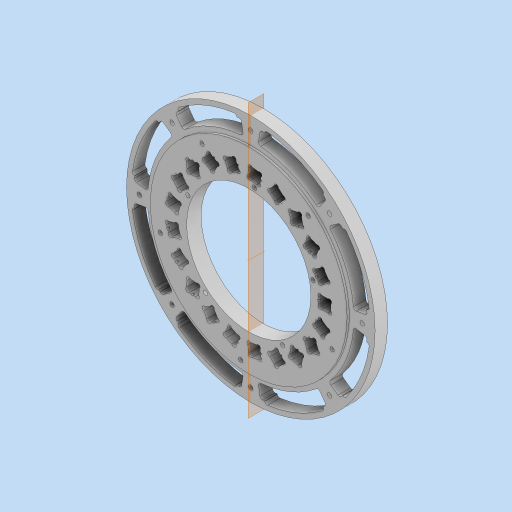
# Autodesk Inventor part: Ring_0
Saved by Autodesk Inventor 2024.2 (Build 282272000, 272)
## iProperties
Created: 2025-04-23
Part Number: Ring_0
Material: Generic
Document SubType Name: Modeling
Designer: 23661194
Density: 1 g/cm^3
Appearance: Default
Author: 23661194
Autodesk Inventor part; units mm, degrees
ref_plane "XZ Plane" through (0, 0, 0) normal (0, 1, 0) x (-1, 0, 0)
ref_plane "XY Plane" through (0, 0, 0) normal (0, 0, 1) x (1, 0, 0)
sketch "Shim Tray Slot_1" plane through (0, 0, 0) normal (0, 0, 1) x (1, 0, 0)
  line L0 (30.092, 109.0254) -> (29.9458, 108.3375)
  line L1 (33.5758, 105.3229) -> (31.6829, 97.1237)
  line L2 (-33.5758, 105.3229) -> (-31.6821, 97.1202)
  line L3 (-30.092, 109.0254) -> (-29.9458, 108.3375)
  arc A0 (-32.2001, 107.689) -> (-33.5758, 105.3229) centre (-31.6271, 105.7728) ccw
  arc A1 (29.147, 95.658) -> (-29.1504, 95.657) centre (0, 0) ccw
  arc A2 (28.6337, 111.3782) -> (-28.6337, 111.3782) centre (0, 0) ccw
  arc A3 (-29.9458, 108.3375) -> (-32.2001, 107.689) centre (0, 0) ccw
  arc A4 (32.2001, 107.689) -> (29.9458, 108.3375) centre (0, 0) ccw
  arc A5 (-28.6337, 111.3782) -> (-30.092, 109.0254) centre (-28.1357, 109.4412) ccw
  arc A6 (-31.6821, 97.1202) -> (-29.1504, 95.657) centre (-29.7334, 97.5701) ccw
  arc A7 (29.147, 95.658) -> (31.6829, 97.1237) centre (29.7309, 97.5743) ccw
  arc A8 (33.5758, 105.3229) -> (32.2001, 107.689) centre (31.6271, 105.7728) ccw
  arc A9 (30.092, 109.0254) -> (28.6337, 111.3782) centre (28.1357, 109.4412) ccw
  line L4 (0, 0) -> (0, 107.5)
  arc A10 (33.9656, 105.2329) -> (32.3146, 108.0722) centre (31.6271, 105.7728) ccw
  line L5 (33.9656, 105.2329) -> (32.0726, 97.0337)
  arc A11 (29.0304, 95.2754) -> (32.0726, 97.0337) centre (29.7309, 97.5743) ccw
  arc A12 (29.0304, 95.2754) -> (-29.0338, 95.2743) centre (0, 0) ccw
  arc A13 (-32.0718, 97.0302) -> (-29.0338, 95.2743) centre (-29.7334, 97.5701) ccw
  line L6 (-32.0718, 97.0302) -> (-33.9656, 105.2329)
  arc A14 (-32.3146, 108.0722) -> (-33.9656, 105.2329) centre (-31.6271, 105.7728) ccw
  arc A15 (-30.4152, 108.6221) -> (-32.3146, 108.0722) centre (0, 0) ccw
  line L7 (-30.4152, 108.6221) -> (-30.4833, 108.9422)
  arc A16 (-28.7333, 111.7656) -> (-30.4833, 108.9422) centre (-28.1357, 109.4412) ccw
  arc A17 (28.7333, 111.7656) -> (-28.7333, 111.7656) centre (0, 0) ccw
  arc A18 (30.4833, 108.9422) -> (28.7333, 111.7656) centre (28.1357, 109.4412) ccw
  line L8 (30.4833, 108.9422) -> (30.4152, 108.6221)
  arc A19 (32.3146, 108.0722) -> (30.4152, 108.6221) centre (0, 0) ccw
  dimension "d182" = 22.5
  dimension "d191" = 0.4
  measures "d191" radial gap between concentric circles of A2 A17
sketch "Sketch1" plane through (0, 0, 0) normal (0, 0, 1) x (1, 0, 0)
  circle A0 centre (0, 0) radius 60
  circle A1 centre (0, 0) radius 120
  circle A2 centre (0, 0) radius 95
  dimension "d0" = 120
  dimension "d1" = 240
  dimension "d2" = 190
  constraints: 3 centre point, 3 coincident
  measures "d0" diameter of A0
  measures "d1" diameter of A1
  measures "d2" diameter of A2
extrude "Extrusion1" add sketch "Sketch1" along normal blind 12 contours A1 | A2
extrude "Extrusion2" add sketch "Sketch1" along normal blind 14 contours A2
sketch "Sketch2" plane through (0, 0, 14) normal (0, 0, 1) x (1, 0, 0)
  circle A0 centre (0, 0) radius 73.485
  line L0 (73.485, 0) -> (0, 0)
  line L1 (70.2203, 21.6601) -> (0, 0)
  line L2 (60.7162, 41.3956) -> (0, 0)
  line L3 (45.8171, 57.4529) -> (0, 0)
  line L4 (26.8471, 68.4053) -> (0, 0)
  line L5 (5.4915, 73.2795) -> (0, 0)
  line L6 (-16.352, 71.6426) -> (0, 0)
  line L7 (-36.7425, 63.6399) -> (0, 0)
  line L8 (-53.8683, 49.9825) -> (0, 0)
  line L9 (-66.2077, 31.8839) -> (0, 0)
  line L10 (-72.6642, 10.9524) -> (0, 0)
  line L11 (-72.6642, -10.9524) -> (0, 0)
  line L12 (-66.2077, -31.8839) -> (0, 0)
  line L13 (-53.8683, -49.9825) -> (0, 0)
  line L14 (-36.7425, -63.6399) -> (0, 0)
  line L15 (-16.352, -71.6426) -> (0, 0)
  line L16 (5.4915, -73.2795) -> (0, 0)
  line L17 (26.8471, -68.4053) -> (0, 0)
  line L18 (45.8171, -57.4529) -> (0, 0)
  line L19 (60.7162, -41.3956) -> (0, 0)
  line L20 (70.2203, -21.6601) -> (0, 0)
  line L21 (-168, 0) -> (168, 0) projected
  line L22 (79.425, 5.94) -> (67.545, 5.94)
  line L23 (67.545, 5.94) -> (67.545, -5.94)
  line L24 (67.545, -5.94) -> (79.425, -5.94)
  line L25 (79.425, -5.94) -> (79.425, 5.94)
  line L26 (79.425, 5.94) -> (67.545, -5.94) construction
  line L27 (67.545, 5.94) -> (79.425, -5.94) construction
  circle A1 centre (73.485, 0) radius 2
  circle A2 centre (68.958, -4.527) radius 2.1
  circle A3 centre (78.012, -4.527) radius 2.1
  circle A4 centre (78.012, 4.527) radius 2.1
  circle A5 centre (68.958, 4.527) radius 2.1
  circle A6 centre (67.185, 0) radius 0.75
  line L28 (67.185, 0) -> (73.485, 0)
  line L29 (71.782, 29.9141) -> (61.9663, 23.2218)
  line L30 (61.9663, 23.2218) -> (68.6585, 13.4061)
  line L31 (68.6585, 13.4061) -> (78.4742, 20.0983)
  line L32 (78.4742, 20.0983) -> (71.782, 29.9141)
  line L33 (71.782, 29.9141) -> (68.6585, 13.4061) construction
  line L34 (61.9663, 23.2218) -> (78.4742, 20.0983) construction
  circle A7 centre (70.2203, 21.6601) radius 2
  circle A8 centre (69.03, 15.3696) radius 2.1
  circle A9 centre (76.5108, 20.4699) radius 2.1
  circle A10 centre (71.4105, 27.9506) radius 2.1
  circle A11 centre (63.9297, 22.8503) radius 2.1
  circle A12 centre (65.015, 18.1112) radius 0.75
  line L35 (65.015, 18.1112) -> (70.2203, 21.6601)
  line L36 (57.3569, 49.0951) -> (53.0166, 38.0363)
  line L37 (53.0166, 38.0363) -> (64.0754, 33.6961)
  line L38 (64.0754, 33.6961) -> (68.4157, 44.7548)
  line L39 (68.4157, 44.7548) -> (57.3569, 49.0951)
  line L40 (57.3569, 49.0951) -> (64.0754, 33.6961) construction
  line L41 (53.0166, 38.0363) -> (68.4157, 44.7548) construction
  circle A13 centre (60.7162, 41.3956) radius 2
  circle A14 centre (63.2763, 35.5276) radius 2.1
  circle A15 centre (66.5841, 43.9557) radius 2.1
  circle A16 centre (58.156, 47.2635) radius 2.1
  circle A17 centre (54.8482, 38.8354) radius 2.1
  circle A18 centre (58.4145, 35.5311) radius 0.75
  line L42 (58.4145, 35.5311) -> (60.7162, 41.3956)
  line L43 (38.7043, 61.9222) -> (41.3479, 50.34)
  line L44 (41.3479, 50.34) -> (52.93, 52.9836)
  line L45 (52.93, 52.9836) -> (50.2864, 64.5657)
  line L46 (50.2864, 64.5657) -> (38.7043, 61.9222)
  line L47 (38.7043, 61.9222) -> (52.93, 52.9836) construction
  line L48 (41.3479, 50.34) -> (50.2864, 64.5657) construction
  circle A19 centre (45.8171, 57.4529) radius 2
  circle A20 centre (51.238, 54.0467) radius 2.1
  circle A21 centre (49.2233, 62.8737) radius 2.1
  circle A22 centre (40.3963, 60.859) radius 2.1
  circle A23 centre (42.411, 52.032) radius 2.1
  circle A24 centre (47.219, 51.3108) radius 0.75
  line L49 (47.219, 51.3108) -> (45.8171, 57.4529)
  line L50 (18.4525, 68.0912) -> (27.1612, 60.0107)
  line L51 (27.1612, 60.0107) -> (35.2416, 68.7194)
  line L52 (35.2416, 68.7194) -> (26.533, 76.7998)
  line L53 (26.533, 76.7998) -> (18.4525, 68.0912)
  line L54 (18.4525, 68.0912) -> (35.2416, 68.7194) construction
  line L55 (27.1612, 60.0107) -> (26.533, 76.7998) construction
  circle A25 centre (26.8471, 68.4053) radius 2
  circle A26 centre (33.2448, 68.6446) radius 2.1
  circle A27 centre (26.6077, 74.8029) radius 2.1
  circle A28 centre (20.4494, 68.1659) radius 2.1
  circle A29 centre (27.0865, 62.0076) radius 2.1
  circle A30 centre (31.4653, 64.1202) radius 0.75
  line L56 (31.4653, 64.1202) -> (26.8471, 68.4053)
  line L57 (-1.2674, 68.2912) -> (10.4799, 66.5206)
  line L58 (10.4799, 66.5206) -> (12.2505, 78.2679)
  line L59 (12.2505, 78.2679) -> (0.5032, 80.0385)
  line L60 (0.5032, 80.0385) -> (-1.2674, 68.2912)
  line L61 (-1.2674, 68.2912) -> (12.2505, 78.2679) construction
  line L62 (10.4799, 66.5206) -> (0.5032, 80.0385) construction
  circle A31 centre (5.4915, 73.2795) radius 2
  circle A32 centre (10.6427, 77.0812) radius 2.1
  circle A33 centre (1.6898, 78.4307) radius 2.1
  circle A34 centre (0.3404, 69.4778) radius 2.1
  circle A35 centre (9.2933, 68.1284) radius 2.1
  circle A36 centre (11.7212, 72.3406) radius 0.75
  line L63 (11.7212, 72.3406) -> (5.4915, 73.2795)
  line L64 (-19.1264, 63.7136) -> (-8.4229, 68.8681)
  line L65 (-8.4229, 68.8681) -> (-13.5775, 79.5716)
  line L66 (-13.5775, 79.5716) -> (-24.281, 74.4171)
  line L67 (-24.281, 74.4171) -> (-19.1264, 63.7136)
  line L68 (-19.1264, 63.7136) -> (-13.5775, 79.5716) construction
  line L69 (-8.4229, 68.8681) -> (-24.281, 74.4171) construction
  circle A37 centre (-16.352, 71.6426) radius 2
  circle A38 centre (-14.2375, 77.6855) radius 2.1
  circle A39 centre (-22.3948, 73.7571) radius 2.1
  circle A40 centre (-18.4664, 65.5997) radius 2.1
  circle A41 centre (-10.3091, 69.5281) radius 2.1
  circle A42 centre (-10.6758, 74.376) radius 0.75
  line L70 (-10.6758, 74.376) -> (-16.352, 71.6426)
  line L71 (-34.5683, 55.5257) -> (-28.6283, 65.8141)
  line L72 (-28.6283, 65.8141) -> (-38.9167, 71.7541)
  line L73 (-38.9167, 71.7541) -> (-44.8567, 61.4657)
  line L74 (-44.8567, 61.4657) -> (-34.5683, 55.5257)
  line L75 (-34.5683, 55.5257) -> (-38.9167, 71.7541) construction
  line L76 (-28.6283, 65.8141) -> (-44.8567, 61.4657) construction
  circle A43 centre (-36.7425, 63.6399) radius 2
  circle A44 centre (-38.3995, 69.8239) radius 2.1
  circle A45 centre (-42.9265, 61.9829) radius 2.1
  circle A46 centre (-35.0855, 57.4559) radius 2.1
  circle A47 centre (-30.5585, 65.2969) radius 2.1
  circle A48 centre (-33.5925, 69.0958) radius 0.75
  line L77 (-33.5925, 69.0958) -> (-36.7425, 63.6399)
  line L78 (-47.501, 44.503) -> (-48.3888, 56.3498)
  line L79 (-48.3888, 56.3498) -> (-60.2356, 55.462)
  line L80 (-60.2356, 55.462) -> (-59.3478, 43.6152)
  line L81 (-59.3478, 43.6152) -> (-47.501, 44.503)
  line L82 (-47.501, 44.503) -> (-60.2356, 55.462) construction
  line L83 (-48.3888, 56.3498) -> (-59.3478, 43.6152) construction
  circle A49 centre (-53.8683, 49.9825) radius 2
  circle A50 centre (-58.721, 54.1585) radius 2.1
  circle A51 centre (-58.0444, 45.1298) radius 2.1
  circle A52 centre (-49.0157, 45.8065) radius 2.1
  circle A53 centre (-49.6923, 54.8351) radius 2.1
  circle A54 centre (-54.3391, 56.2649) radius 0.75
  line L84 (-54.3391, 56.2649) -> (-53.8683, 49.9825)
  line L85 (-57.8601, 30.9434) -> (-65.2671, 40.2316)
  line L86 (-65.2671, 40.2316) -> (-74.5553, 32.8245)
  line L87 (-74.5553, 32.8245) -> (-67.1482, 23.5363)
  line L88 (-67.1482, 23.5363) -> (-57.8601, 30.9434)
  line L89 (-57.8601, 30.9434) -> (-74.5553, 32.8245) construction
  line L90 (-65.2671, 40.2316) -> (-67.1482, 23.5363) construction
  circle A55 centre (-66.2077, 31.8839) radius 2
  circle A56 centre (-72.5696, 32.6008) radius 2.1
  circle A57 centre (-66.9245, 25.5221) radius 2.1
  circle A58 centre (-59.8458, 31.1671) radius 2.1
  circle A59 centre (-65.4909, 38.2458) radius 2.1
  circle A60 centre (-70.1357, 36.8095) radius 0.75
  line L91 (-70.1357, 36.8095) -> (-66.2077, 31.8839)
  line L92 (-65.2373, 14.8776) -> (-76.5895, 18.3793)
  line L93 (-76.5895, 18.3793) -> (-80.0912, 7.0271)
  line L94 (-80.0912, 7.0271) -> (-68.739, 3.5254)
  line L95 (-68.739, 3.5254) -> (-65.2373, 14.8776)
  line L96 (-65.2373, 14.8776) -> (-80.0912, 7.0271) construction
  line L97 (-76.5895, 18.3793) -> (-68.739, 3.5254) construction
  circle A61 centre (-72.6642, 10.9524) radius 2
  circle A62 centre (-78.3245, 7.9608) radius 2.1
  circle A63 centre (-69.6727, 5.2921) radius 2.1
  circle A64 centre (-67.004, 13.9439) radius 2.1
  circle A65 centre (-75.6558, 16.6126) radius 2.1
  circle A66 centre (-78.6843, 12.8093) radius 0.75
  line L98 (-78.6843, 12.8093) -> (-72.6642, 10.9524)
  line L99 (-68.739, -3.5254) -> (-80.0912, -7.0271)
  line L100 (-80.0912, -7.0271) -> (-76.5895, -18.3793)
  line L101 (-76.5895, -18.3793) -> (-65.2373, -14.8776)
  line L102 (-65.2373, -14.8776) -> (-68.739, -3.5254)
  line L103 (-68.739, -3.5254) -> (-76.5895, -18.3793) construction
  line L104 (-80.0912, -7.0271) -> (-65.2373, -14.8776) construction
  circle A67 centre (-72.6642, -10.9524) radius 2
  circle A68 centre (-75.6558, -16.6126) radius 2.1
  circle A69 centre (-67.004, -13.9439) radius 2.1
  circle A70 centre (-69.6727, -5.2921) radius 2.1
  circle A71 centre (-78.3245, -7.9608) radius 2.1
  circle A72 centre (-78.6843, -12.8093) radius 0.75
  line L105 (-78.6843, -12.8093) -> (-72.6642, -10.9524)
  line L106 (-67.1482, -23.5363) -> (-74.5553, -32.8245)
  line L107 (-74.5553, -32.8245) -> (-65.2671, -40.2316)
  line L108 (-65.2671, -40.2316) -> (-57.8601, -30.9434)
  line L109 (-57.8601, -30.9434) -> (-67.1482, -23.5363)
  line L110 (-67.1482, -23.5363) -> (-65.2671, -40.2316) construction
  line L111 (-74.5553, -32.8245) -> (-57.8601, -30.9434) construction
  circle A73 centre (-66.2077, -31.8839) radius 2
  circle A74 centre (-65.4909, -38.2458) radius 2.1
  circle A75 centre (-59.8458, -31.1671) radius 2.1
  circle A76 centre (-66.9245, -25.5221) radius 2.1
  circle A77 centre (-72.5696, -32.6008) radius 2.1
  circle A78 centre (-70.1357, -36.8095) radius 0.75
  line L112 (-70.1357, -36.8095) -> (-66.2077, -31.8839)
  line L113 (-59.3478, -43.6152) -> (-60.2356, -55.462)
  line L114 (-60.2356, -55.462) -> (-48.3888, -56.3498)
  line L115 (-48.3888, -56.3498) -> (-47.501, -44.503)
  line L116 (-47.501, -44.503) -> (-59.3478, -43.6152)
  line L117 (-59.3478, -43.6152) -> (-48.3888, -56.3498) construction
  line L118 (-60.2356, -55.462) -> (-47.501, -44.503) construction
  circle A79 centre (-53.8683, -49.9825) radius 2
  circle A80 centre (-49.6923, -54.8351) radius 2.1
  circle A81 centre (-49.0157, -45.8065) radius 2.1
  circle A82 centre (-58.0444, -45.1298) radius 2.1
  circle A83 centre (-58.721, -54.1585) radius 2.1
  circle A84 centre (-54.3391, -56.2649) radius 0.75
  line L119 (-54.3391, -56.2649) -> (-53.8683, -49.9825)
  line L120 (-44.8567, -61.4657) -> (-38.9167, -71.7541)
  line L121 (-38.9167, -71.7541) -> (-28.6283, -65.8141)
  line L122 (-28.6283, -65.8141) -> (-34.5683, -55.5257)
  line L123 (-34.5683, -55.5257) -> (-44.8567, -61.4657)
  line L124 (-44.8567, -61.4657) -> (-28.6283, -65.8141) construction
  line L125 (-38.9167, -71.7541) -> (-34.5683, -55.5257) construction
  circle A85 centre (-36.7425, -63.6399) radius 2
  circle A86 centre (-30.5585, -65.2969) radius 2.1
  circle A87 centre (-35.0855, -57.4559) radius 2.1
  circle A88 centre (-42.9265, -61.9829) radius 2.1
  circle A89 centre (-38.3995, -69.8239) radius 2.1
  circle A90 centre (-33.5925, -69.0958) radius 0.75
  line L126 (-33.5925, -69.0958) -> (-36.7425, -63.6399)
  line L127 (-24.281, -74.4171) -> (-13.5775, -79.5716)
  line L128 (-13.5775, -79.5716) -> (-8.4229, -68.8681)
  line L129 (-8.4229, -68.8681) -> (-19.1264, -63.7136)
  line L130 (-19.1264, -63.7136) -> (-24.281, -74.4171)
  line L131 (-24.281, -74.4171) -> (-8.4229, -68.8681) construction
  line L132 (-13.5775, -79.5716) -> (-19.1264, -63.7136) construction
  circle A91 centre (-16.352, -71.6426) radius 2
  circle A92 centre (-10.3091, -69.5281) radius 2.1
  circle A93 centre (-18.4664, -65.5997) radius 2.1
  circle A94 centre (-22.3948, -73.7571) radius 2.1
  circle A95 centre (-14.2375, -77.6855) radius 2.1
  circle A96 centre (-10.6758, -74.376) radius 0.75
  line L133 (-10.6758, -74.376) -> (-16.352, -71.6426)
  line L134 (0.5032, -80.0385) -> (12.2505, -78.2679)
  line L135 (12.2505, -78.2679) -> (10.4799, -66.5206)
  line L136 (10.4799, -66.5206) -> (-1.2674, -68.2912)
  line L137 (-1.2674, -68.2912) -> (0.5032, -80.0385)
  line L138 (0.5032, -80.0385) -> (10.4799, -66.5206) construction
  line L139 (12.2505, -78.2679) -> (-1.2674, -68.2912) construction
  circle A97 centre (5.4915, -73.2795) radius 2
  circle A98 centre (9.2933, -68.1284) radius 2.1
  circle A99 centre (0.3404, -69.4778) radius 2.1
  circle A100 centre (1.6898, -78.4307) radius 2.1
  circle A101 centre (10.6427, -77.0812) radius 2.1
  circle A102 centre (11.7212, -72.3406) radius 0.75
  line L140 (11.7212, -72.3406) -> (5.4915, -73.2795)
  line L141 (26.533, -76.7998) -> (35.2416, -68.7194)
  line L142 (35.2416, -68.7194) -> (27.1612, -60.0107)
  line L143 (27.1612, -60.0107) -> (18.4525, -68.0912)
  line L144 (18.4525, -68.0912) -> (26.533, -76.7998)
  line L145 (26.533, -76.7998) -> (27.1612, -60.0107) construction
  line L146 (35.2416, -68.7194) -> (18.4525, -68.0912) construction
  circle A103 centre (26.8471, -68.4053) radius 2
  circle A104 centre (27.0865, -62.0076) radius 2.1
  circle A105 centre (20.4494, -68.1659) radius 2.1
  circle A106 centre (26.6077, -74.8029) radius 2.1
  circle A107 centre (33.2448, -68.6446) radius 2.1
  circle A108 centre (31.4653, -64.1202) radius 0.75
  line L147 (31.4653, -64.1202) -> (26.8471, -68.4053)
  line L148 (50.2864, -64.5657) -> (52.93, -52.9836)
  line L149 (52.93, -52.9836) -> (41.3479, -50.34)
  line L150 (41.3479, -50.34) -> (38.7043, -61.9222)
  line L151 (38.7043, -61.9222) -> (50.2864, -64.5657)
  line L152 (50.2864, -64.5657) -> (41.3479, -50.34) construction
  line L153 (52.93, -52.9836) -> (38.7043, -61.9222) construction
  circle A109 centre (45.8171, -57.4529) radius 2
  circle A110 centre (42.411, -52.032) radius 2.1
  circle A111 centre (40.3963, -60.859) radius 2.1
  circle A112 centre (49.2233, -62.8737) radius 2.1
  circle A113 centre (51.238, -54.0467) radius 2.1
  circle A114 centre (47.219, -51.3108) radius 0.75
  line L154 (47.219, -51.3108) -> (45.8171, -57.4529)
  line L155 (68.4157, -44.7548) -> (64.0754, -33.6961)
  line L156 (64.0754, -33.6961) -> (53.0166, -38.0363)
  line L157 (53.0166, -38.0363) -> (57.3569, -49.0951)
  line L158 (57.3569, -49.0951) -> (68.4157, -44.7548)
  line L159 (68.4157, -44.7548) -> (53.0166, -38.0363) construction
  line L160 (64.0754, -33.6961) -> (57.3569, -49.0951) construction
  circle A115 centre (60.7162, -41.3956) radius 2
  circle A116 centre (54.8482, -38.8354) radius 2.1
  circle A117 centre (58.156, -47.2635) radius 2.1
  circle A118 centre (66.5841, -43.9557) radius 2.1
  circle A119 centre (63.2763, -35.5276) radius 2.1
  circle A120 centre (58.4145, -35.5311) radius 0.75
  line L161 (58.4145, -35.5311) -> (60.7162, -41.3956)
  line L162 (78.4742, -20.0983) -> (68.6585, -13.4061)
  line L163 (68.6585, -13.4061) -> (61.9663, -23.2218)
  line L164 (61.9663, -23.2218) -> (71.782, -29.9141)
  line L165 (71.782, -29.9141) -> (78.4742, -20.0983)
  line L166 (78.4742, -20.0983) -> (61.9663, -23.2218) construction
  line L167 (68.6585, -13.4061) -> (71.782, -29.9141) construction
  circle A121 centre (70.2203, -21.6601) radius 2
  circle A122 centre (63.9297, -22.8503) radius 2.1
  circle A123 centre (71.4105, -27.9506) radius 2.1
  circle A124 centre (76.5108, -20.4699) radius 2.1
  circle A125 centre (69.03, -15.3696) radius 2.1
  circle A126 centre (65.015, -18.1112) radius 0.75
  line L168 (65.015, -18.1112) -> (70.2203, -21.6601)
  point P0 (69.3309, -28.243)
  point P1 (73.4531, -27.463)
  point P2 (76.8031, -22.5494)
  point P3 (76.0232, -18.4272)
  point P4 (71.1096, -15.0772)
  point P5 (66.9874, -15.8572)
  point P6 (63.6374, -20.7708)
  point P7 (64.4173, -24.8929)
  point P8 (54.1004, -40.7978)
  point P9 (56.2731, -46.3336)
  point P10 (60.1183, -48.0113)
  point P11 (65.6542, -45.8386)
  point P12 (67.3319, -41.9934)
  point P13 (65.1592, -36.4575)
  point P14 (61.314, -34.7799)
  point P15 (55.7781, -36.9525)
  point P16 (39.3644, -59.03)
  point P17 (41.5964, -62.5823)
  point P18 (47.3943, -63.9056)
  point P19 (50.9466, -61.6736)
  point P20 (52.2699, -55.8757)
  point P21 (50.0378, -52.3235)
  point P22 (44.24, -51.0002)
  point P23 (40.6877, -53.2322)
  point P24 (24.5152, -74.6252)
  point P25 (28.7076, -74.7821)
  point P26 (33.067, -70.7371)
  point P27 (33.2239, -66.5447)
  point P28 (29.1789, -62.1853)
  point P29 (24.9866, -62.0285)
  point P30 (20.6271, -66.0734)
  point P31 (20.4703, -70.2658)
  point P32 (1.666, -67.849)
  point P33 (-0.8253, -71.2246)
  point P34 (0.0611, -77.1051)
  point P35 (3.4366, -79.5964)
  point P36 (9.3171, -78.71)
  point P37 (11.8084, -75.3345)
  point P38 (10.922, -69.4539)
  point P39 (7.5465, -66.9627)
  point P40 (-16.4537, -65.0007)
  point P41 (-20.4136, -66.3863)
  point P42 (-22.9938, -71.7443)
  point P43 (-21.6082, -75.7042)
  point P44 (-16.2502, -78.2845)
  point P45 (-12.2903, -76.8989)
  point P46 (-9.7101, -71.5408)
  point P47 (-11.0957, -67.581)
  point P48 (-37.1374, -57.0089)
  point P49 (-42.2876, -59.9824)
  point P50 (-43.3734, -64.0348)
  point P51 (-40.4, -69.185)
  point P52 (-36.3476, -70.2708)
  point P53 (-31.1974, -67.2973)
  point P54 (-30.1116, -63.245)
  point P55 (-33.085, -58.0948)
  point P56 (-47.7227, -47.4612)
  point P57 (-50.4593, -44.2813)
  point P58 (-56.3896, -43.8369)
  point P59 (-59.5695, -46.5734)
  point P60 (-60.0139, -52.5038)
  point P61 (-57.2774, -55.6837)
  point P62 (-51.3471, -56.1281)
  point P63 (-48.1671, -53.3916)
  point P64 (-64.8289, -25.3859)
  point P65 (-68.9978, -25.8557)
  point P66 (-72.7057, -30.5052)
  point P67 (-72.236, -34.6741)
  point P68 (-67.5865, -38.382)
  point P69 (-63.4176, -37.9122)
  point P70 (-59.7097, -33.2627)
  point P71 (-60.1794, -29.0938)
  point P72 (-67.8646, -6.3602)
  point P73 (-71.5737, -4.3998)
  point P74 (-77.2565, -6.1527)
  point P75 (-79.2168, -9.8618)
  point P76 (-77.4639, -15.5446)
  point P77 (-73.7548, -17.5049)
  point P78 (-68.072, -15.752)
  point P79 (-66.1117, -12.0429)
  point P80 (-66.1117, 12.0429)
  point P81 (-68.072, 15.752)
  point P82 (-73.7548, 17.5049)
  point P83 (-77.4639, 15.5446)
  point P84 (-79.2168, 9.8618)
  point P85 (-77.2565, 6.1527)
  point P86 (-71.5737, 4.3998)
  point P87 (-67.8646, 6.3602)
  point P88 (-60.1794, 29.0938)
  point P89 (-59.7097, 33.2627)
  point P90 (-63.4176, 37.9122)
  point P91 (-67.5865, 38.382)
  point P92 (-72.236, 34.6741)
  point P93 (-72.7057, 30.5052)
  point P94 (-68.9978, 25.8557)
  point P95 (-64.8289, 25.3859)
  point P96 (-47.7227, 47.4612)
  point P97 (-48.1671, 53.3916)
  point P98 (-51.3471, 56.1281)
  point P99 (-57.2774, 55.6837)
  point P100 (-60.0139, 52.5038)
  point P101 (-59.5695, 46.5734)
  point P102 (-56.3896, 43.8369)
  point P103 (-50.4593, 44.2813)
  point P104 (-37.1374, 57.0089)
  point P105 (-33.085, 58.0948)
  point P106 (-30.1116, 63.245)
  point P107 (-31.1974, 67.2973)
  point P108 (-36.3476, 70.2708)
  point P109 (-40.4, 69.185)
  point P110 (-43.3734, 64.0348)
  point P111 (-42.2876, 59.9824)
  point P112 (-11.0957, 67.581)
  point P113 (-9.7101, 71.5408)
  point P114 (-12.2903, 76.8989)
  point P115 (-16.2502, 78.2845)
  point P116 (-21.6082, 75.7042)
  point P117 (-22.9938, 71.7443)
  point P118 (-20.4136, 66.3863)
  point P119 (-16.4537, 65.0007)
  point P120 (-0.8253, 71.2246)
  point P121 (1.666, 67.849)
  point P122 (7.5465, 66.9627)
  point P123 (10.922, 69.4539)
  point P124 (11.8084, 75.3345)
  point P125 (9.3171, 78.71)
  point P126 (3.4366, 79.5964)
  point P127 (0.0611, 77.1051)
  point P128 (20.4703, 70.2658)
  point P129 (20.6271, 66.0734)
  point P130 (24.9866, 62.0285)
  point P131 (29.1789, 62.1853)
  point P132 (33.2239, 66.5447)
  point P133 (33.067, 70.7371)
  point P134 (28.7076, 74.7821)
  point P135 (24.5152, 74.6252)
  point P136 (39.3644, 59.03)
  point P137 (40.6877, 53.2322)
  point P138 (44.24, 51.0002)
  point P139 (50.0378, 52.3235)
  point P140 (52.2699, 55.8757)
  point P141 (50.9466, 61.6736)
  point P142 (47.3943, 63.9056)
  point P143 (41.5964, 62.5823)
  point P144 (65.1592, 36.4575)
  point P145 (67.3319, 41.9934)
  point P146 (65.6542, 45.8386)
  point P147 (60.1183, 48.0113)
  point P148 (56.2731, 46.3336)
  point P149 (54.1004, 40.7978)
  point P150 (55.7781, 36.9525)
  point P151 (61.314, 34.7799)
  point P152 (64.4173, 24.8929)
  point P153 (63.6374, 20.7708)
  point P154 (66.9874, 15.8572)
  point P155 (71.1096, 15.0772)
  point P156 (76.0232, 18.4272)
  point P157 (76.8031, 22.5494)
  point P158 (73.4531, 27.463)
  point P159 (69.3309, 28.243)
  point P160 (70.5115, 5.94)
  point P161 (67.545, 2.9735)
  point P162 (67.545, -2.9735)
  point P163 (70.5115, -5.94)
  point P164 (76.4585, -5.94)
  point P165 (79.425, -2.9735)
  point P166 (79.425, 2.9735)
  point P167 (76.4585, 5.94)
  dimension "d7" = 146.97
  dimension "d119" = -34.286
  dimension "d120" = -68.571
  dimension "d121" = -102.857
  dimension "d122" = -137.143
  dimension "d123" = -171.429
  dimension "d124" = -205.714
  dimension "d125" = -240
  dimension "d126" = -274.286
  dimension "d127" = -308.571
  dimension "d128" = -342.857
  dimension "d129" = -17.143
  dimension "d130" = -51.429
  dimension "d131" = -85.714
  dimension "d132" = -120
  dimension "d133" = -154.286
  dimension "d134" = -188.571
  dimension "d135" = -222.857
  dimension "d136" = -257.143
  dimension "d137" = -291.429
  dimension "d138" = -325.714
  dimension "d10" = 360
  dimension "d118" = 0
  constraints: 42 end point, 1 coincident, 1 horizontal, 1 horizontal alignment, 88 other
  measures "d118" vertical extent of L0
extrude "Extrusion3" cut sketch "Sketch2" against normal blind 12 contours L0 A1 A0 | L21 A1 A0 | A0 A1 L0 | A0 A1 L21 | A1 L0 A6 L23 A5 L22 A0 | A0 L22 A4 L25 L21 A1 | A1 L21 L25 A3 L24 A0 | A0 L24 A2 L23 A6 L0 A1 | A6 L23 L0 | L0 L23 A6 | L31 A8 L30 A12 L35 A7 A0 | A0 A7 L29 A10 L32 A9 L31 | A4 L25 L22 | L22 L25 A4 | A5 L23 L22 | L22 L23 A5 | L162 A124 L165 A123 L164 A0 A121 | A0 A121 L168 A126 L163 A125 L162 | A2 L23 L24 | L24 L23 A2 | A3 L25 L24 | L24 L25 A3 | A7 L35 A0 | A0 A7 | A8 L30 L31 | L31 L30 A8 | A9 L32 L31 | L31 L32 A9 | A121 A0 | A0 L168 A121 | A124 L165 L162 | L162 L165 A124 | A125 L163 L162 | L162 L163 A125 | L1 A7 A0 | L35 A7 L1 | L35 A12 L30 L1 A7 | A0 A121 L20 | L20 A121 L168 | A121 L20 L163 A126 L168 | A7 L1 L30 A11 L29 A0 | L35 L30 A12 | A12 L30 L35 | A10 L29 L32 | L32 L29 A10 | A0 L164 A122 L163 L20 A121 | L168 L163 A126 | A126 L163 L168 | A123 L164 L165 | L165 L164 A123 | A17 L36 L37 L2 | L2 L37 A17 | A23 L43 L3 | L3 L43 L44 A23 | L50 A28 L53 A0 A25 L4 | L4 A25 L56 A30 L51 A29 L50 | L57 A34 L60 A0 A31 L5 | L5 A31 L63 A36 L58 A35 L57 | L64 A40 L67 A0 A37 L6 | L6 A37 A0 L65 A41 L64 | A46 L74 L71 L7 | L7 L71 A46 | A52 L81 L8 | L8 L81 L78 A52 | L88 A57 A0 A55 L9 | L9 A55 A0 L85 A58 L88 | L95 A63 L94 A0 A61 L10 | L10 A61 A0 L92 A64 L95 | L102 A69 L101 A0 A67 L11 | L11 A67 A0 L99 A70 L102 | L109 A75 L108 A0 A73 L12 | L12 A73 A0 A76 L109 | A81 L115 L116 L13 | L13 L116 A81 | A87 L122 L14 | L14 L122 L123 A87 | L129 A92 L128 A0 A91 L15 | L15 A91 A0 L130 A93 L129 | L136 A98 L135 A102 L140 A97 L16 | L16 A97 A0 L137 A99 L136 | L143 A104 L142 A108 L147 A103 L17 | L17 A103 A0 L144 A105 L143 | A110 L149 L150 L18 | L18 L150 A110 | A116 L156 L19 | L19 L156 L157 A116 | A11 L29 L30 | L30 L29 A11 | L37 L36 A17 L2 | L2 A17 L37 | L36 A16 A0 A13 L2 A17 | A17 L2 A13 L42 A18 L37 | L43 A23 L3 | L3 A23 L44 L43 | L43 A22 A0 A19 L3 A23 | A23 L3 A19 L49 A24 L44 | A25 A0 L4 | L4 L56 A25 | A28 L53 L50 | L50 L53 A28 | A29 L51 L50 | L50 L51 A29 | A31 A0 L5 | L5 L63 A31 | A34 L60 L57 | L57 L60 A34 | A35 L58 L57 | L57 L58 A35 | A37 A0 L6 | L6 A0 A37 | A40 L67 L64 | L64 L67 A40 | A41 L65 L64 | L64 L65 A41 | L71 L74 A46 L7 | L7 A46 L71 | L74 A45 A0 A43 L7 A46 | L81 A52 L8 | L8 A52 L78 L81 | L81 A51 A0 A49 L8 A52 | A55 A0 L9 | L9 A0 A55 | A57 A0 L87 L88 | L88 L87 A0 A57 | A58 L85 L88 | L88 L85 A58 | A61 A0 L10 | L10 A0 A61 | A63 L94 L95 | L95 L94 A63 | A64 L92 L95 | L95 L92 A64 | A67 A0 L11 | L11 A0 A67 | A69 L101 L102 | L102 L101 A69 | A70 L99 L102 | L102 L99 A70 | A73 A0 L12 | L12 A0 A73 | A75 L108 L109 | L109 L108 A75 | A76 A0 L106 L109 | L109 L106 A0 A76 | L116 L115 A81 L13 | L13 A81 L116 | A81 L13 A79 A0 A82 L116 | L122 A87 L14 | L14 A87 L123 L122 | A87 L14 A85 A0 A88 L123 | A91 A0 L15 | L15 A0 A91 | A92 L128 L129 | L129 L128 A92 | A93 L130 L129 | L129 L130 A93 | A97 L140 L16 | L16 A0 A97 | A98 L135 L136 | L136 L135 A98 | A99 L137 L136 | L136 L137 A99 | A103 L147 L17 | L17 A0 A103 | A104 L142 L143 | L143 L142 A104 | A105 L144 L143 | L143 L144 A105 | L150 L149 A110 L18 | L18 A110 L150 | L149 A114 L154 A109 L18 A110 | A110 L18 A109 A0 A111 L150 | L156 A116 L19 | L19 A116 L157 L156 | L156 A120 L161 A115 L19 A116 | A116 L19 A115 A0 A117 L157 | A122 L164 L163 | L163 L164 A122 | L94 A62 L93 A66 L98 A61 A0 | A0 A67 L105 A72 L100 A71 L99 | A14 L37 L38 A0 | A0 L38 A14 | A119 L155 A0 | A0 L155 L156 A119 | A16 A0 L36 | L36 A0 A16 | A18 L42 L37 | A22 A0 L46 L43 | L43 L46 A0 A22 | A24 L49 L44 | A0 A25 | A0 A25 L56 | A0 L53 A27 L52 A26 L51 A25 | A25 A0 L51 A30 L56 | A0 A31 | A0 A31 L63 | A0 L60 A33 L59 A32 L58 A36 A31 | A31 A0 A36 L63 | L70 A37 A0 | A0 A37 L70 | A0 L67 A39 L66 A38 L65 A42 L70 A37 | L7 A43 A0 A47 L71 A46 | A45 A0 L74 | L74 A0 A45 | L8 A49 A0 A53 L78 A52 | A51 A0 L81 | L81 A0 A51 | L91 A55 A0 | A0 A55 L91 | A0 A57 L87 A56 L86 A60 L91 A55 | A57 L87 A0 | L98 A61 A0 | A0 A61 L98 | L105 A67 A0 | A0 A67 L105 | L112 A73 A0 | A0 A73 L112 | A73 L112 A78 L107 A77 L106 A76 A0 | A0 L106 A76 | A81 L115 A80 A0 A79 L13 | A82 A0 L116 | L116 A0 A82 | A87 L122 A86 A0 A85 L14 | A88 A0 L123 | L123 A0 A88 | L133 A91 A0 | A0 A91 L133 | A91 L133 A96 L128 A95 L127 A94 L130 A0 | A0 A97 | L140 A97 A0 | L140 A102 A0 A97 | A97 A0 A102 L135 A101 L134 A100 L137 | A0 A103 | L147 A103 A0 | L147 A108 L142 A0 A103 | A103 A0 L142 A107 L141 A106 L144 | L149 L154 A114 | A111 A0 L151 L150 | L150 L151 A0 A111 | L156 L161 A120 | A117 A0 L157 | L157 A0 A117 | A62 L93 L94 | L94 L93 A62 | A71 L100 L99 | L99 L100 A71 | L38 L37 A14 A0 | A0 A14 L38 | L37 A18 L42 A13 A0 A14 | L155 A119 A0 | A0 A119 L156 L155 | A119 A0 A115 L161 A120 L156 | A13 A0 L2 | L2 L42 A13 | L36 L39 A16 A0 | A0 A16 L39 L36 | A16 L39 A15 L38 A14 A0 A13 | L42 A18 L37 | A19 A0 L3 | L3 L49 A19 | A22 L46 A0 | A22 L46 A21 L45 A20 A0 A19 | A0 L46 A22 | L49 A24 L44 | L49 A19 A0 A20 L44 A24 | L56 L51 A30 | A30 L51 L56 | L63 L58 A36 | A36 A0 L58 L63 | A37 L70 A42 L65 A0 | A43 A0 L7 | L7 A0 A43 | A47 A0 L72 L71 | L71 L72 A0 A47 | L74 L73 A45 A0 | A0 A45 L73 L74 | A45 L73 A44 L72 A48 L77 A43 A0 | A49 A0 L8 | L8 A0 A49 | L81 L80 A51 A0 | A0 A51 L80 L81 | A53 A0 L78 | L78 A0 A53 | A55 L91 A60 L86 A59 L85 A0 | A0 L87 A57 | A0 A61 L98 A66 L93 A65 L92 | A0 L101 A68 L100 A72 L105 A67 | A0 L108 A74 L107 A78 L112 A73 | A76 L106 A0 | A79 A0 L13 | L13 A0 A79 | A80 A0 L115 | L115 A0 A80 | L116 L113 A82 A0 | A0 A82 L113 L116 | A85 A0 L14 | L14 A0 A85 | A86 A0 L121 L122 | L122 L121 A0 A86 | L123 L120 A88 A0 | A0 A88 L120 L123 | A0 A85 L126 A90 L121 A89 L120 A88 | A0 L128 A96 L133 A91 | L140 L135 A0 A102 | A102 L135 L140 | L147 L142 A108 | A108 L142 L147 | A109 L154 L18 | L18 A0 A109 | L149 A114 L154 | A114 L149 A113 A0 A109 L154 | A111 L151 A0 | A0 A109 A113 L148 A112 L151 A111 | A0 L151 A111 | A115 L161 L19 | L19 A0 A115 | L156 A120 L161 | L157 L158 A117 A0 | A0 A117 L158 L157 | A0 A115 A119 L155 A118 L158 A117 | A0 A13 | A0 A13 L42 | A20 L44 A0 | A0 L44 L45 A20 | A0 A19 | A0 A19 L49 | A27 L52 L53 | L53 L52 A27 | A36 L58 A0 | A33 L59 L60 | L60 L59 A33 | L70 L65 A42 | A42 L65 L70 | A0 L72 A47 | A39 L66 L67 | L67 L66 A39 | L77 A43 A0 | A0 A43 L77 | A47 L72 A0 | A0 A43 L77 A48 L72 A47 | A0 L78 L79 A53 | L84 A49 A0 | A0 A49 L84 | A0 A51 L80 A50 L79 A54 L84 A49 | A0 A53 L79 L78 | A0 A49 L84 A54 L79 A53 | L91 L86 A60 | A60 L86 L91 | A65 L93 L92 | L92 L93 A65 | A56 L86 L87 | L87 L86 A56 | A59 L86 L85 | L85 L86 A59 | L98 L93 A66 | A66 L93 L98 | L105 L100 A72 | A72 L100 L105 | A68 L100 L101 | L101 L100 A68 | L112 L107 A78 | A78 L107 L112 | A74 L107 L108 | L108 L107 A74 | A77 L107 L106 | L106 L107 A77 | L119 A79 A0 | A0 A79 L119 | A79 L119 A84 L114 A83 L113 A82 A0 | L115 L114 A80 A0 | A0 A80 L114 L115 | A80 L114 A84 L119 A79 A0 | L126 A85 A0 | A0 A85 L126 | A86 L121 A90 L126 A85 A0 | A0 L121 A86 | L133 L128 A96 | A96 L128 L133 | A86 L121 A0 | A94 L127 L130 | L130 L127 A94 | A0 L135 A102 | A100 L134 L137 | L137 L134 A100 | A106 L141 L144 | L144 L141 A106 | A0 A109 | L154 A109 A0 | A0 A115 | L161 A115 A0 | A113 L148 L149 A0 | A0 L149 A113 | A15 L39 L38 | L38 L39 A15 | A118 L158 L155 | L155 L158 A118 | L44 A20 A0 | A0 A20 L45 L44 | A26 L52 L51 | L51 L52 A26 | A21 L45 L46 | L46 L45 A21 | A44 L72 L73 | L73 L72 A44 | A50 L79 L80 | L80 L79 A50 | A83 L114 L113 | L113 L114 A83 | A89 L121 L120 | L120 L121 A89 | A107 L141 L142 | L142 L141 A107 | L149 A0 A113 | A112 L148 L151 | L151 L148 A112 | L149 L148 A113 A0 | A32 L59 L58 | L58 L59 A32 | A38 L66 L65 | L65 L66 A38 | A48 L77 L72 | A48 L72 L77 | A54 L84 L79 | A54 L79 L84 | L119 L114 A84 | A84 L114 L119 | L126 L121 A90 | A90 L121 L126 | A95 L127 L128 | L128 L127 A95 | A101 L134 L135 | L135 L134 A101 picked at (67.5888, -0.4081) picked at (67.5888, 0.4081) picked at (11.3962, 72.8737) picked at (11.3962, -72.8737)
extrude "Extrusion4" cut sketch "Sketch2" against normal blind 2 contours A6 L23 L0 | L0 L23 A6 | L23 A6 L0 | L0 A6 L23 | L35 L30 A12 | A12 L30 L35 | A12 L30 | L168 L163 A126 | A126 L163 L168 | L163 A126 | A18 L42 L37 | L37 A18 | A24 L49 L44 | L44 A24 | A114 L149 | L149 L154 A114 | A120 L156 | L156 L161 A120 | L42 A18 L37 | L49 A24 L44 | L56 L51 A30 | A30 L51 L56 | L51 A30 | L63 L58 A36 | A36 A0 L58 L63 | L58 A0 A36 | L140 L135 A0 A102 | A102 L135 L140 | A102 A0 L135 | L147 L142 A108 | A108 L142 L147 | A108 L142 | L149 A114 L154 | L156 A120 L161 | A0 L58 A36 | A36 L58 A0 | L70 L65 A42 | A42 L65 L70 | L65 A42 | L91 L86 A60 | A60 L86 L91 | L98 L93 A66 | A66 L93 L98 | L105 L100 A72 | A72 L100 L105 | L112 L107 A78 | A78 L107 L112 | L133 L128 A96 | A96 L128 L133 | A96 L128 | A0 L135 A102 | A102 L135 A0 | A66 L93 | L100 A72 | A60 L86 | L107 A78 | A48 L77 L72 | L72 A48 | A48 L72 L77 | A54 L84 L79 | L79 A54 | A54 L79 L84 | L119 L114 A84 | A84 L114 L119 | A84 L114 | L126 L121 A90 | A90 L121 L126 | A90 L121
extrude "Extrusion5" cut sketch "Sketch2" against normal through all contours L0 A1 A0 | L21 A1 A0 | A0 A1 L0 | A0 A1 L21 | A7 L35 A0 | A0 A7 | A121 A0 | A0 L168 A121 | L1 A7 A0 | L35 A7 L1 | A0 A121 L20 | L20 A121 L168 | A25 A0 L4 | L4 L56 A25 | A31 A0 L5 | L5 L63 A31 | A37 A0 L6 | L6 A0 A37 | A55 A0 L9 | L9 A0 A55 | A61 A0 L10 | L10 A0 A61 | A67 A0 L11 | L11 A0 A67 | A73 A0 L12 | L12 A0 A73 | A91 A0 L15 | L15 A0 A91 | A97 L140 L16 | L16 A0 A97 | A103 L147 L17 | L17 A0 A103 | A0 A25 | A0 A25 L56 | A0 A31 | A0 A31 L63 | L70 A37 A0 | A0 A37 L70 | L91 A55 A0 | A0 A55 L91 | L98 A61 A0 | A0 A61 L98 | L105 A67 A0 | A0 A67 L105 | L112 A73 A0 | A0 A73 L112 | L133 A91 A0 | A0 A91 L133 | A0 A97 | L140 A97 A0 | A0 A103 | L147 A103 A0 | A13 A0 L2 | L2 L42 A13 | A19 A0 L3 | L3 L49 A19 | A43 A0 L7 | L7 A0 A43 | A49 A0 L8 | L8 A0 A49 | A79 A0 L13 | L13 A0 A79 | A85 A0 L14 | L14 A0 A85 | A109 L154 L18 | L18 A0 A109 | A115 L161 L19 | L19 A0 A115 | A0 A13 | A0 A13 L42 | A0 A19 | A0 A19 L49 | L77 A43 A0 | A0 A43 L77 | L84 A49 A0 | A0 A49 L84 | L119 A79 A0 | A0 A79 L119 | L126 A85 A0 | A0 A85 L126 | A0 A109 | L154 A109 A0 | A0 A115 | L161 A115 A0
sketch "Sketch3" plane through (0, 0, 12) normal (0, 0, 1) x (1, 0, 0)
  circle A0 centre (0, 0) radius 107.5
  circle A1 centre (0, 107.5) radius 2.15
  circle A2 centre (-76.014, 76.014) radius 2.15
  circle A3 centre (-107.5, 0) radius 2.15
  circle A4 centre (-76.014, -76.014) radius 2.15
  circle A5 centre (0, -107.5) radius 2.15
  circle A6 centre (76.014, -76.014) radius 2.15
  circle A7 centre (107.5, 0) radius 2.15
  circle A8 centre (76.014, 76.014) radius 2.15
  dimension "d145" = 215
  dimension "d146" = 4.3
  dimension "d149" = 360
  constraints: 8 centre point, 1 coincident, 1 vertical alignment, 19 other
  measures "d146" diameter of A1
extrude "Extrusion6" cut sketch "Sketch3" against normal through all contours A0 A7 | A0 A7 | A8 A0 | A0 A8 | A6 A0 | A0 A6 | A1 A0 | A0 A1 | A5 A0 | A0 A5 | A2 A0 | A0 A2 | A4 A0 | A0 A4 | A3 A0 | A0 A3
sketch "Sketch4" plane through (0, 0, 14) normal (0, 0, 1) x (1, 0, 0)
  circle A0 centre (0, 0) radius 63.75
  circle A1 centre (0, 0) radius 87.5
  line L0 (0, 0) -> (5.5562, 63.5074)
  line L1 (0, 168) -> (0, -168) projected
  circle A2 centre (5.5562, 63.5074) radius 2.1
  circle A3 centre (-58.6822, 24.9091) radius 2.1
  circle A4 centre (-41.8238, -48.1127) radius 2.1
  circle A5 centre (32.8337, -54.6444) radius 2.1
  circle A6 centre (62.1161, 14.3406) radius 2.1
  line L2 (0, 0) -> (57.4052, 66.0371)
  circle A7 centre (57.4052, 66.0371) radius 2.1
  circle A8 centre (-45.0658, 75.0021) radius 2.1
  circle A9 centre (-85.2574, -19.6832) radius 2.1
  circle A10 centre (-7.6261, -87.167) radius 2.1
  circle A11 centre (80.5442, -34.189) radius 2.1
  dimension "d153" = 127.5
  dimension "d159" = 175
  dimension "d160" = 5
  dimension "d161" = 4.2
  dimension "d172" = 360
  dimension "d174" = 41
  dimension "d175" = 4.2
  dimension "d178" = 360
  constraints: 10 centre point, 4 coincident, 4 end point, 28 other
  measures "d160" angle of L1 L0
  measures "d161" diameter of A2
  measures "d174" angle of L1 L2
  measures "d175" diameter of A7
extrude "Extrusion7" cut sketch "Sketch4" against normal blind 8 contours A6 A0 | A0 A6 | A5 A0 | A0 A5 | A2 L0 A0 | A0 A2 | A7 A1 L2 | L2 A1 A7 | A4 A0 | A0 A4 | L0 A2 A0 | A1 A7 | A10 A1 | A1 A10 | A11 A1 | A1 A11 | A3 A0 | A0 A3 | A8 A1 | A1 A8 | A9 A1 | A1 A9
sketch "Sketch5" plane through (0, 0, 12) normal (0, 0, 1) x (1, 0, 0)
  line L0 (0, 168) -> (0, -168) projected
  line L1 (69.5236, 89.2106) -> (69.1253, 88.631)
  line L2 (71.3254, 84.4568) -> (66.4388, 77.6061)
  line L3 (9.2853, 110.1546) -> (7.8959, 101.8516)
  line L4 (13.9208, 112.2421) -> (13.7927, 111.5505)
  arc A0 (11.4618, 111.8141) -> (9.2853, 110.1546) centre (11.2579, 109.8245) ccw
  arc A1 (63.5351, 77.2224) -> (9.6749, 99.5309) centre (0, 0) ccw
  arc A2 (69.0767, 91.9424) -> (16.1685, 113.8577) centre (0, 0) ccw
  arc A3 (13.7927, 111.5505) -> (11.4618, 111.8141) centre (0, 0) ccw
  arc A4 (70.9598, 87.1692) -> (69.1253, 88.631) centre (0, 0) ccw
  arc A5 (16.1685, 113.8577) -> (13.9208, 112.2421) centre (15.8873, 111.8776) ccw
  arc A6 (7.8959, 101.8516) -> (9.6749, 99.5309) centre (9.8684, 101.5215) ccw
  arc A7 (63.5351, 77.2224) -> (66.4388, 77.6061) centre (64.8079, 78.7694) ccw
  arc A8 (71.3254, 84.4568) -> (70.9598, 87.1692) centre (69.6971, 85.6182) ccw
  arc A9 (69.5236, 89.2106) -> (69.0767, 91.9424) centre (67.8754, 90.3434) ccw
  line L5 (0, 0) -> (41.1385, 99.317)
  arc A10 (71.651, 84.2245) -> (71.2123, 87.4794) centre (69.6971, 85.6182) ccw
  line L6 (71.651, 84.2245) -> (66.7645, 77.3738)
  arc A11 (63.2809, 76.9135) -> (66.7645, 77.3738) centre (64.8079, 78.7694) ccw
  arc A12 (63.2809, 76.9135) -> (9.6362, 99.1328) centre (0, 0) ccw
  arc A13 (7.5013, 101.9176) -> (9.6362, 99.1328) centre (9.8684, 101.5215) ccw
  line L7 (7.5013, 101.9176) -> (8.8908, 110.2206)
  arc A14 (11.5026, 112.212) -> (8.8908, 110.2206) centre (11.2579, 109.8245) ccw
  arc A15 (13.4679, 111.9931) -> (11.5026, 112.212) centre (0, 0) ccw
  line L8 (13.4679, 111.9931) -> (13.5275, 112.3149)
  arc A16 (16.2248, 114.2537) -> (13.5275, 112.3149) centre (15.8873, 111.8776) ccw
  arc A17 (69.317, 92.2622) -> (16.2248, 114.2537) centre (0, 0) ccw
  arc A18 (69.8533, 88.9841) -> (69.317, 92.2622) centre (67.8754, 90.3434) ccw
  line L9 (69.8533, 88.9841) -> (69.6679, 88.7143)
  arc A19 (71.2123, 87.4794) -> (69.6679, 88.7143) centre (0, 0) ccw
  point P0 (70.9598, 87.1692)
  dimension "d183" = 22.5
  constraints: 1 other
extrude "Extrusion9" cut sketch "Sketch5" against normal through all contours L1 A4 A8 L2 A7 A1 A6 L3 A0 A3 L4 A5 A2 A9 | L6 A11 A12 A13 L7 A14 A15 L8 A16 A17 A18 L9 A19 A10
pattern_circular "Circular Pattern2" count 8 over 360 about axis through (0, 0, -10) along (0, 0, 1) of "Extrusion9"
sketch "Block2" plane through (0, 0, 0) normal (0, 0, 1) x (1, 0, 0)
  line L0 (83.1381, 5.88) -> (71.258, 5.88)
  line L1 (71.258, 5.88) -> (71.258, -6)
  line L2 (71.258, -6) -> (83.1381, -6)
  line L3 (83.1381, -6) -> (83.1381, 5.88)
  line L4 (83.1381, 5.88) -> (71.258, -6) construction
  line L5 (71.258, 5.88) -> (83.1381, -6) construction
  circle A0 centre (77.198, -0.06) radius 2
  circle A1 centre (72.671, -4.587) radius 2.1
  circle A2 centre (81.725, -4.587) radius 2.1
  circle A3 centre (81.725, 4.467) radius 2.1
  circle A4 centre (72.671, 4.467) radius 2.1
  circle A5 centre (70.898, -0.06) radius 0.75
  line L6 (70.898, -0.06) -> (77.198, -0.06)
  dimension "d13" = 11.88
  dimension "d15" = 4.2
  dimension "d12" = 11.88
  dimension "d14" = 4
  dimension "d16" = 1.413
  dimension "d17" = 360
  dimension "d18" = 1.5
  dimension "d19" = 6.3
  constraints: 6 end point, 2 centre point, 2 coincident, 2 midpoint, 1 horizontal, 1 point on line, 21 other
  measures "d12" distance of L5.end L4.end
  measures "d14" diameter of A0
  measures "d18" diameter of A5
  measures "d19" distance of L6.end L6.start
body "Solid1"
